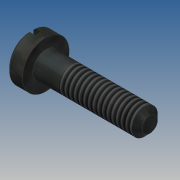
# Autodesk Inventor part: Schlitzschraube_ra8846s
Saved by Autodesk Inventor 2021 (Build 250183000, 183)
## iProperties
Created: 2020-11-17
Part Number: Schlitzschraube_ra8846s
Material: Stahl
Document SubType Name: Modeling
Designer: Ricardo A
Density: 7.85 g/cm^3
Appearance: Platte
Description: Motor_Teil4_schraube
Mass: 0.517812 g
Surface Area: 1.31567 cm^2
Volume: 0.0659633 cm^3
Author: Sander
Revision Number: Rev00
Autodesk Inventor part; units mm, degrees
ref_plane "YZ-Ebene" through (0, 0, 0) normal (1, 0, 0) x (0, 1, 0)
ref_plane "XZ-Ebene" through (0, 0, 0) normal (0, 1, 0) x (-1, 0, 0)
ref_plane "XY-Ebene" through (0, 0, 0) normal (0, 0, 1) x (1, 0, 0)
sketch "Skizze1" plane through (0, 0, 0) normal (0, 0, 1) x (1, 0, 0)
  line L0 (-2.3, 0) -> (13.8, 0) projected
  line L1 (0, -0.45) -> (0, 2.7) projected
  line L2 (0, 2.25) -> (1.5, 2.25)
  line L3 (1.5, 2.25) -> (1.5, 1.25)
  line L4 (1.5, 1.25) -> (11.5, 1.25)
  line L5 (11.5, 1.25) -> (11.5, 0)
  point P0 (0, 0)
  dimension "d0" = 1.5
  dimension "d1" = 10
  dimension "d2" = 1.25
  dimension "d3" = 2.25
  constraints: 8 end point, 4 perpendicular, 2 point on line
  measures "d0" distance of L2.start L2.end
  measures "d1" distance of L3.end L4.end
  measures "d2" distance of L4.end L5.end
  measures "d3" distance from line of L2 point (0, 0)
revolve "Umdrehung1" add sketch "Skizze1" angle 360 about axis through (-10, 0, 0) along (1, 0, 0)
sketch "Skizze2" plane through (0, 0, 0) normal (-1, 0, 0) x (0, 0, 1)
  circle A0 centre (0, 0) radius 2.25 projected
  line L0 (-3.15, 0) -> (3.15, 0) projected
  line L1 (2.2299, 0.3) -> (-2.2299, 0.3)
  line L2 (-2.2299, -0.3) -> (2.2299, -0.3)
  dimension "d5" = 0.6
  constraints: 4 end point, 4 point on circle, 1 horizontal, 1 parallel, 1 other
  measures "d5" distance between parallel lines of L2 L1
extrude "Extrusion1" cut sketch "Skizze2" against normal blind 0.8 contours L0 A0 L1 | A0 L2 L0
chamfer "Fase1" distance 0.5 angle 45 1 edges at (11.5, -1.25, 0)
thread "Gewinde1" size "M2.5x0.45" class "6g" standard "ISO Metric profile" length 7
chamfer "Fase2" distance 0.25 angle 45 3 edges at (0, -2.25, 0) (0, 1.6937, 1.4811) (0, 1.6937, -1.4811)
